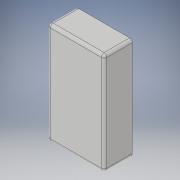
# Autodesk Inventor part: Table foot
Saved by Autodesk Inventor 2018 (Build 220112000, 112)
## iProperties
Created: 2018-05-16
Part Number: Table foot
Material: Generic
Document SubType Name: Modeling
Designer: 4070439
Density: 1 g/cm^3
Appearance: Default
Author: 4070439
## iProperties of the stored document Table foot_3DPrint.ipt
Created: 2018-05-16
Part Number: Table foot_3DPrint
Material: Generic
Document SubType Name: Modeling
Designer: 4070439
Density: 1 g/cm^3
Appearance: Default
Author: 4070439
Autodesk Inventor part; units mm, degrees
ref_plane "YZ Plane" through (0, 0, 0) normal (1, 0, 0) x (0, 1, 0)
ref_plane "XZ Plane" through (0, 0, 0) normal (0, 1, 0) x (-1, 0, 0)
ref_plane "XY Plane" through (0, 0, 0) normal (0, 0, 1) x (1, 0, 0)
sketch "Sketch1" plane through (0, 0, 0) normal (0, 0, 1) x (1, 0, 0)
  line L0 (-25.4, -50.8) -> (25.4, -50.8)
  line L1 (25.4, -50.8) -> (25.4, 50.8)
  line L2 (25.4, 50.8) -> (-25.4, 50.8)
  line L3 (-25.4, 50.8) -> (-25.4, -50.8)
  line L4 (-25.4, -50.8) -> (25.4, 50.8) construction
  line L5 (25.4, -50.8) -> (-25.4, 50.8) construction
  point P0 (0, 0)
  dimension "d0" = 50.8
  dimension "d1" = 101.6
  constraints: 12 end point, 2 midpoint, 2 parallel, 1 horizontal, 1 perpendicular
  measures "d0" distance of L1.end L2.end
  measures "d1" distance of L2.end L0.start
extrude "Extrusion1" add sketch "Sketch1" along normal blind 6.35
sketch "Sketch2" plane through (25.4, -50.8, 0) normal (1, 0, 0) x (0, 0, -1)
  line L0 (-6.35, 0) -> (-6.35, 101.6) projected
  line L1 (-6.35, 101.6) -> (0, 101.6)
  line L2 (0, 101.6) -> (0, 0)
  line L3 (0, 0) -> (-6.35, 0)
  line L4 (-6.35, 0) -> (-6.35, 101.6)
  point P0 (0, 50.8)
  constraints: 8 end point, 2 parallel, 1 horizontal, 1 perpendicular
extrude "Extrusion2" add sketch "Sketch2" along normal blind 6.35
sketch "Sketch3" plane through (-25.4, -50.8, 0) normal (-1, 0, 0) x (0, 0, 1)
  point P0 (0, 50.8)
sketch "Sketch4" plane through (-25.4, -50.8, 0) normal (-1, 0, 0) x (0, 0, 1)
  line L0 (6.35, 101.6) -> (6.35, 0) projected
  line L1 (0, 0) -> (6.35, 0) projected
  line L2 (6.35, 101.6) -> (0, 101.6)
  line L3 (0, 101.6) -> (0, 0)
  line L4 (0, 0) -> (6.35, 0)
  line L5 (6.35, 0) -> (6.35, 101.6)
  point P0 (0, 50.8)
  constraints: 8 end point, 2 parallel, 1 horizontal, 1 perpendicular
extrude "Extrusion3" add sketch "Sketch4" along normal blind 6.35
sketch "Sketch5" plane through (31.75, -50.8, 0) normal (0, -1, 0) x (1, 0, 0)
  line L0 (-63.5, 0) -> (-63.5, 6.35) projected
  line L1 (0, 6.35) -> (0, 0) projected
  line L2 (-63.5, 0) -> (0, 0)
  line L3 (0, 0) -> (0, 6.35)
  line L4 (0, 6.35) -> (-63.5, 6.35)
  line L5 (-63.5, 6.35) -> (-63.5, 0)
  point P0 (-31.75, 0)
  constraints: 8 end point, 2 parallel, 1 horizontal, 1 perpendicular
extrude "Extrusion4" add sketch "Sketch5" along normal blind 6.35
sketch "Sketch6" plane through (31.75, 50.8, 6.35) normal (0, 1, 0) x (1, 0, 0)
  line L0 (-63.5, 0) -> (0, 0) projected
  line L1 (-63.5, 6.35) -> (0, 6.35) projected
  line L2 (-63.5, 0) -> (0, 0)
  line L3 (0, 0) -> (0, 6.35)
  line L4 (0, 6.35) -> (-63.5, 6.35)
  line L5 (-63.5, 6.35) -> (-63.5, 0)
  point P0 (-31.75, 6.35)
  constraints: 8 end point, 2 parallel, 1 horizontal, 1 perpendicular
extrude "Extrusion5" add sketch "Sketch6" along normal blind 6.35
sketch "Sketch7" plane through (0, 0, 0) normal (0, 0, -1) x (-1, 0, 0)
  line L0 (31.75, -57.15) -> (31.75, 57.15) projected
  line L1 (31.75, -57.15) -> (25.4, -57.15)
  line L2 (25.4, -57.15) -> (25.4, 57.15)
  line L3 (25.4, 57.15) -> (31.75, 57.15)
  line L4 (31.75, 57.15) -> (31.75, -57.15)
  line L5 (-31.75, -57.15) -> (-25.4, -57.15)
  line L6 (-25.4, -57.15) -> (-25.4, 57.15)
  line L7 (-25.4, 57.15) -> (-31.75, 57.15)
  line L8 (-31.75, 57.15) -> (-31.75, -57.15)
  line L9 (25.4, -57.15) -> (-25.4, -57.15)
  line L10 (-25.4, -57.15) -> (-25.4, -50.8)
  line L11 (-25.4, -50.8) -> (25.4, -50.8)
  line L12 (25.4, -50.8) -> (25.4, -57.15)
  line L13 (25.4, 57.15) -> (-25.4, 57.15)
  line L14 (-25.4, 57.15) -> (-25.4, 50.8)
  line L15 (-25.4, 50.8) -> (25.4, 50.8)
  line L16 (25.4, 50.8) -> (25.4, 57.15)
  point P0 (0, 0)
  dimension "d12" = 6.35
  dimension "d13" = 114.3
  dimension "d14" = 6.35
  dimension "d15" = 114.3
  dimension "d16" = 50.8
  dimension "d17" = 6.35
  dimension "d18" = 6.35
  dimension "d19" = 50.8
  constraints: 32 end point, 8 parallel, 4 horizontal, 4 perpendicular
  measures "d12" distance of L2.end L3.end
  measures "d13" distance of L1.end L2.end
  measures "d14" distance of L6.end L7.end
  measures "d15" distance of L5.end L6.end
  measures "d16" distance of L10.end L11.end
  measures "d17" distance of L9.end L10.end
  measures "d18" distance of L13.end L14.end
  measures "d19" distance of L14.end L15.end
extrude "Extrusion6" add sketch "Sketch7" along normal blind 25.4 contours L5 L8 L7 L6
sketch "Sketch8" plane through (25.4, -57.15, 0) normal (-1, 0, 0) x (0, 0, 1)
  line L0 (6.35, 0) -> (-25.4, 0) projected
  line L1 (-25.4, 0) -> (0, 0)
  line L2 (0, 0) -> (0, 6.35)
  line L3 (0, 6.35) -> (-25.4, 6.35)
  line L4 (-25.4, 6.35) -> (-25.4, 0)
  point P0 (0, 57.15)
  dimension "d22" = 25.4
  dimension "d23" = 6.35
  constraints: 8 end point, 2 parallel, 1 horizontal, 1 perpendicular
  measures "d22" distance of L2.end L3.end
  measures "d23" distance of L1.end L2.end
extrude "Extrusion7" add sketch "Sketch8" along normal blind 57.15
sketch "Sketch9" plane through (25.4, 57.15, -25.4) normal (-1, 0, 0) x (0, 0, 1)
  line L0 (0, 0) -> (0, -114.3) projected
  line L1 (0, 0) -> (25.4, 0)
  line L2 (25.4, 0) -> (25.4, -6.35)
  line L3 (25.4, -6.35) -> (0, -6.35)
  line L4 (0, -6.35) -> (0, 0)
  point P0 (25.4, -57.15)
  dimension "d26" = 25.4
  dimension "d27" = 6.35
  constraints: 8 end point, 2 parallel, 1 horizontal, 1 perpendicular
  measures "d26" distance of L2.end L3.end
  measures "d27" distance of L1.end L2.end
extrude "Extrusion8" add sketch "Sketch9" along normal blind 57.15
sketch "Sketch10" plane through (25.4, -50.8, 0) normal (0, 1, 0) x (1, 0, 0)
  line L0 (0, 25.4) -> (-57.15, 25.4) projected
  line L1 (-57.15, 25.4) -> (-50.8, 25.4)
  line L2 (-50.8, 25.4) -> (-50.8, 0)
  line L3 (-50.8, 0) -> (-57.15, 0)
  line L4 (-57.15, 0) -> (-57.15, 25.4)
  point P0 (-25.4, 0)
  dimension "d30" = 6.35
  dimension "d31" = 25.4
  constraints: 8 end point, 2 parallel, 1 horizontal, 1 perpendicular
  measures "d30" distance of L2.end L3.end
  measures "d31" distance of L1.end L2.end
extrude "Extrusion9" add sketch "Sketch10" along normal blind 101.6
fillet "Fillet1" radius 3.175 1 edges at (0, -57.15, 6.35)
fillet "Fillet2" radius 3.175 3 edges at (-31.75, 1.5875, 6.35) (-31.75, -56.2201, 5.4201) (-31.75, -57.15, -11.1125)
fillet "Fillet3" radius 3.175 3 edges at (1.5875, 57.15, 6.35) (-30.8201, 57.15, 5.4201) (-31.75, 57.15, -11.1125)
fillet "Fillet4" radius 3.175 5 edges at (31.75, 0, 6.35) (31.75, 56.2201, 5.4201) (31.75, 57.15, -11.1125) (31.75, -56.2201, 5.4201) (31.75, -57.15, -11.1125)
body "Solid1"
